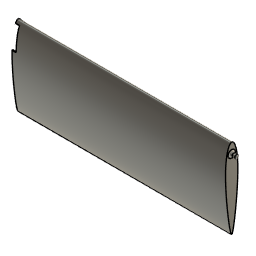
ailerons v11 (Autodesk Fusion 360 design; units mm, degrees)
Autodesk Fusion 360 part; units mm, degrees
note: some values were not read from the file. Set by a fixed rule: which sketch regions a step uses.
sketch "Sketch1" plane through (0, 0, 0) normal (1, 0, 0) x (0, 1, 0)
  spline S0 degree 5 poles (0, 0) (-0.0984, 0) (-0.2953, 0.2081) (-0.6031, 1.1448) (-1.0883, 3.5986) (-1.7768, 8.3639) (-2.4496, 14.3583) (-2.9457, 20.9396) (-3.1157, 27.3952) (-2.7821, 32.7537) (-2.0096, 36.5171) (-1.004, 38.6653) (0, 39.3389) (1.004, 38.6653) (2.0096, 36.5171) (2.7821, 32.7537) (3.1157, 27.3952) (2.9457, 20.9396) (2.4496, 14.3583) (1.7768, 8.3639) (1.0883, 3.5986) (0.6031, 1.1448) (0.2953, 0.2081) (0.0984, 0) (0, 0) knots 0 0 0 0 0 0 0.05 0.1 0.15 0.2 0.25 0.3 0.35 0.4 0.45 0.5 0.55 0.6 0.65 0.7 0.75 0.8 0.85 0.9 0.95 1 1 1 1 1 1
  line L0 (-3, 16) -> (-3, 36)
  line L1 (3, 36) -> (3, 16)
  line L2 (-1.5, 39) -> (1.5, 39)
  line L3 (0.5, 0) -> (-0.5, 0)
  point P0 (-3, 26)
  point P1 (0, 39)
  point P2 (3, 26)
  dimension "d1" = 26
  dimension "d2" = 13
  dimension "d4" = 6
  dimension "d5" = 20
  dimension "d6" = 1
  dimension "d7" = 3
  constraint coincident S0.start S0.end
  constraint midpoint P0 L0
  constraint vertical L0
  constraint midpoint P2 L1
  constraint vertical L1
  constraint midpoint P1 L2
  constraint horizontal L2
  constraint midpoint S0.start L3
  constraint horizontal L3
  constraint horizontal P0 P2
  constraint vertical S0.start P1
  constraint equal L0 L1
  measures "d1" distance of S0.start P0
  measures "d2" vertical distance of P0 P1
  measures "d4" distance of P0 P2
  measures "d5" distance of L1.start L1.end
  measures "d6" distance of L3.start L3.end
  measures "d7" distance of L2.start L2.end
extrude "Extrude1" add sketch "Sketch1" along normal blind 104
sketch "Sketch2" plane through (0, 0, 0) normal (-1, 0, 0) x (0, -1, 0)
  spline S0 degree 5 poles (0, 0) (0.0984, 0) (0.2953, 0.2081) (0.6031, 1.1448) (1.0883, 3.5986) (1.7768, 8.3639) (2.4496, 14.3583) (2.9457, 20.9396) (3.1157, 27.3952) (2.7821, 32.7537) (2.0096, 36.5171) (1.004, 38.6653) (0, 39.3389) (-1.004, 38.6653) (-2.0096, 36.5171) (-2.7821, 32.7537) (-3.1157, 27.3952) (-2.9457, 20.9396) (-2.4496, 14.3583) (-1.7768, 8.3639) (-1.0883, 3.5986) (-0.6031, 1.1448) (-0.2953, 0.2081) (-0.0984, 0) (0, 0) knots 0 0 0 0 0 0 0.05 0.1 0.15 0.2 0.25 0.3 0.35 0.4 0.45 0.5 0.55 0.6 0.65 0.7 0.75 0.8 0.85 0.9 0.95 1 1 1 1 1 1
  circle A0 centre (0, 34) radius 3.65
  circle A1 centre (0, 20) radius 2.25
  line L0 (2.2475, 19.8944) -> (2.8, 31.6585)
  line L1 (-2.2475, 19.8944) -> (-2.8, 31.6585)
  dimension "d10" = 7.3
  dimension "d11" = 4.5
  dimension "d12" = 14
  dimension "d13" = 5.6
  dimension "d14" = 34
  constraint coincident A1 L0.start
  constraint coincident A0 L0.end
  constraint coincident A1 L1.start
  constraint coincident A0 L1.end
  constraint vertical A0.centre A1.centre
  constraint vertical S0.start A1.centre
  constraint tangent A1 L1
  constraint tangent A1 L0
  constraint horizontal L0.end L1.end
  measures "d10" diameter of A0
  measures "d11" diameter of A1
  measures "d12" distance of A0.centre A1.centre
  measures "d13" horizontal distance of L0.end L1.end
  measures "d14" distance of S0.start A0.centre
extrude "Extrude2" cut sketch "Sketch2" against normal blind 2 contours S0 A0 A1 L0 L1 | S0 A0 | A1 picked at (0.1296, 33.0055)
sketch "Sketch3" plane through (104, 0, 0) normal (1, 0, 0) x (0, 1, 0)
  spline S0 degree 5 poles (0, 0) (0.0984, 0) (0.2953, 0.2081) (0.6031, 1.1448) (1.0883, 3.5986) (1.7768, 8.3639) (2.4496, 14.3583) (2.9457, 20.9396) (3.1157, 27.3952) (2.7821, 32.7537) (2.0096, 36.5171) (1.004, 38.6653) (0, 39.3389) (-1.004, 38.6653) (-2.0096, 36.5171) (-2.7821, 32.7537) (-3.1157, 27.3952) (-2.9457, 20.9396) (-2.4496, 14.3583) (-1.7768, 8.3639) (-1.0883, 3.5986) (-0.6031, 1.1448) (-0.2953, 0.2081) (-0.0984, 0) (0, 0) knots -1 -1 -1 -1 -1 -1 -0.95 -0.9 -0.85 -0.8 -0.75 -0.7 -0.65 -0.6 -0.55 -0.5 -0.45 -0.4 -0.35 -0.3 -0.25 -0.2 -0.15 -0.1 -0.05 0 0 0 0 0 0
  circle A0 centre (0, 34) radius 0.8
  dimension "d17" = 1.6
  dimension "d18" = 34
  constraint vertical S0.start A0.centre
  measures "d17" diameter of A0
  measures "d18" distance of S0.start A0.centre
extrude "Extrude3" add sketch "Sketch3" along normal blind 3 contours A0
fillet "Fillet1" radius 1 1 edges at (104, -0.7459, 34.2893)
fillet "Fillet1" radius 0.7 1 edges at (107, -0.7459, 33.7107)
fillet "Fillet1" radius 0.2 4 edges at (1, -1.5285, 37.3146) (1, 1.5285, 37.3146) (1, -2.7837, 31.3111) (1, 2.7837, 31.3111)
